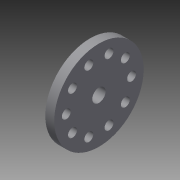
# Autodesk Inventor part: WheelcapTL
Saved by Autodesk Inventor 2015 (Build 190159000, 159)
## iProperties
Created: 2015-01-30
Part Number: WheelcapTL
Material: Generic
Document SubType Name: Modeling
Designer: PLTW-Stu-02
Density: 1 g/cm^3
Appearance: Default
Author: PLTW-Stu-02
Autodesk Inventor part; units mm, degrees
ref_plane "YZ Plane" through (0, 0, 0) normal (1, 0, 0) x (0, 1, 0)
ref_plane "XZ Plane" through (0, 0, 0) normal (0, 1, 0) x (-1, 0, 0)
ref_plane "XY Plane" through (0, 0, 0) normal (0, 0, 1) x (1, 0, 0)
sketch "Sketch1" plane through (0, 0, 0) normal (0, 0, 1) x (1, 0, 0)
  line L0 (12.9819, 11.3591) -> (38.3819, 11.3591)
  line L1 (6.6182, 1.8341) -> (45.5002, 1.8341) construction
  line L2 (12.9819, 11.3591) -> (12.9819, 27.2341)
  line L3 (12.9819, 27.2341) -> (25.6819, 27.2341)
  line L4 (25.6819, 27.2341) -> (25.6819, 65.3341)
  line L5 (25.6819, 65.3341) -> (38.3819, 65.3341)
  line L6 (38.3819, 65.3341) -> (38.3819, 11.3591)
  point P0 (0, 0)
  dimension "d0" = 25.4
  dimension "d1" = 9.525
  dimension "d2" = 15.875
  dimension "d3" = 12.7
  dimension "d4" = 38.1
  constraints: 14 end point, 4 perpendicular, 1 horizontal, 1 parallel, 1 vertical
  measures "d0" distance of L0.start L0.end
  measures "d1" distance between parallel lines of L1 L0
  measures "d2" distance of L0.start L2.end
  measures "d3" distance of L2.end L3.end
  measures "d4" distance of L3.end L4.end
revolve "Revolution2" add sketch "Sketch1" angle 360 about axis through (6.6182, 1.8341, 0) along (1, 0, 0)
sketch "Sketch7" plane through (25.6819, 1.8341, 0) normal (-1, 0, 0) x (0, 0, 1)
  circle A0 centre (0, 0) radius 46.355 construction
  circle A1 centre (0, 0) radius 46.355 construction
  circle A2 centre (0, 0) radius 46.355 construction
  circle A3 centre (0, 0) radius 46.355 construction
  circle A4 centre (0, 0) radius 46.355 construction
  circle A5 centre (0, 0) radius 46.355 construction
  circle A6 centre (0, 0) radius 46.355 construction
  circle A7 centre (0, 0) radius 46.355 construction
  circle A8 centre (0, 0) radius 46.355 construction
  circle A9 centre (0, 0) radius 46.355 construction
  point P0 (0, -1.8341)
  point P1 (-46.355, 0)
  point P2 (-37.502, -27.2468)
  point P3 (-14.3245, -44.0862)
  point P4 (14.3245, -44.0862)
  point P5 (37.502, -27.2468)
  point P6 (46.355, 0)
  point P7 (37.502, 27.2468)
  point P8 (14.3245, 44.0862)
  point P9 (-14.3245, 44.0862)
  point P10 (-37.502, 27.2468)
  dimension "d14" = 92.71
  dimension "d17" = 360
  constraints: 2 coincident, 2 horizontal alignment, 57 other
hole "Hole2" at (25.6819, 1.8341, -46.355) at (25.6819, -25.4126, -37.502) at (25.6819, -42.2521, -14.3245) at (25.6819, -42.2521, 14.3245) at (25.6819, -25.4126, 37.502) at (25.6819, 1.8341, 46.355) at (25.6819, 29.0809, 37.502) at (25.6819, 45.9204, 14.3245) at (25.6819, 45.9204, -14.3245) at (25.6819, 29.0809, -37.502) direction (1, 0, 0) diameter 12.7 end through all
body "Solid2"
